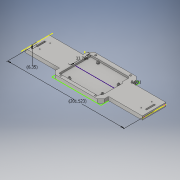
# Autodesk Inventor part: base
Saved by Autodesk Inventor 2016 (Build 200138000, 138)
## iProperties
Created: 2018-02-12
Part Number: base
Material: Generic
Document SubType Name: Modeling
Designer: student
Density: 1 g/cm^3
Appearance: Default
Author: student
Autodesk Inventor part; units mm, degrees
ref_plane "YZ Plane" through (0, 0, 0) normal (1, 0, 0) x (0, 1, 0)
ref_plane "XZ Plane" through (0, 0, 0) normal (0, 1, 0) x (-1, 0, 0)
ref_plane "XY Plane" through (0, 0, 0) normal (0, 0, 1) x (1, 0, 0)
sketch "Sketch1" plane through (0, 0, 0) normal (0, 1, 0) x (-1, 0, 0)
  line L0 (-41.4486, 0) -> (-10.4831, 0)
  line L1 (-10.4831, 0) -> (-10.4831, 53.4636)
  line L2 (-10.4831, 53.4636) -> (-41.4486, 53.4636)
  line L3 (-41.4486, 53.4636) -> (-41.4486, 0)
  line L4 (-79.1688, 53.4636) -> (-87.1698, 53.4636)
  line L5 (-87.1698, 53.4636) -> (-87.1698, 0)
  line L6 (-87.1698, 0) -> (-79.1688, 0)
  line L7 (-79.1688, 0) -> (-79.1688, 53.4636)
  line L8 (-87.1698, 53.4636) -> (-2.487, 53.4636)
  line L9 (-2.487, 53.4636) -> (-2.487, 59.4685)
  line L10 (-2.487, 59.4685) -> (-87.1698, 59.4685)
  line L11 (-87.1698, 59.4685) -> (-87.1698, 53.4636)
  line L12 (-87.1698, 0) -> (-2.487, 0)
  line L13 (-2.487, 0) -> (-2.487, -7.9038)
  line L14 (-2.487, -7.9038) -> (-87.1698, -7.9038)
  line L15 (-87.1698, -7.9038) -> (-87.1698, 0)
  line L16 (-87.1698, -7.9038) -> (-2.487, -7.9038)
  line L17 (-2.487, -7.9038) -> (-2.487, 59.4685)
  line L18 (-2.487, 59.4685) -> (-87.1698, 59.4685)
  line L19 (-87.1698, 59.4685) -> (-87.1698, -7.9038)
  line L20 (-2.487, -7.9038) -> (-2.487, 25.802)
  line L21 (-2.487, 25.802) -> (-2.487, 59.4685)
  point P0 (0, 0)
  dimension "d0" = 8.001
  dimension "d1" = 33.7058
  constraints: 44 end point, 10 parallel, 6 perpendicular, 5 horizontal, 4 point on line
  measures "d0" distance of L6.end L5.end
  measures "d1" distance of L16.end L20.end
extrude "Extrusion1" add sketch "Sketch1" along normal blind 6.35
sketch "Sketch3" plane through (0, 6.35, 0) normal (0, 1, 0) x (1, 0, 0)
  line L0 (10.5148, -0.1125) -> (75.0308, -0.1125) projected
  line L1 (75.0308, -0.1125) -> (76.5548, -1.6365) projected
  line L2 (76.5548, -1.6365) -> (76.5548, -13.003) projected
  line L3 (76.5997, -13.1114) -> (79.0948, -15.6065) projected
  line L4 (79.0948, -15.6065) -> (79.0948, -48.3725) projected
  line L5 (79.0948, -48.3725) -> (76.5997, -50.8676) projected
  line L6 (76.5548, -50.976) -> (76.5548, -53.4525) projected
  line L7 (76.5548, -53.4525) -> (10.5148, -53.4525) projected
  line L8 (10.5148, -53.4525) -> (10.5148, -0.1125) projected
  line L9 (77.3168, -12.7509) -> (77.3168, -1.3209)
  line L10 (77.3168, -1.3209) -> (75.3465, 0.6495)
  line L11 (75.3465, 0.6495) -> (9.7528, 0.6495)
  line L12 (9.7528, 0.6495) -> (9.7528, -54.2145)
  line L13 (9.7528, -54.2145) -> (77.3168, -54.2145)
  line L14 (77.3168, -54.2145) -> (77.3168, -51.2282)
  line L15 (77.3168, -51.2282) -> (79.8568, -48.6882)
  line L16 (79.8568, -48.6882) -> (79.8568, -15.2909)
  line L17 (79.8568, -15.2909) -> (77.3168, -12.7509)
  point P0 (0, 0)
  dimension "d4" = 0.762
  dimension "d5" = 0.762
  dimension "d6" = 0.762
  dimension "d7" = 0.762
  dimension "d8" = 0.762
  dimension "d9" = 0.762
  constraints: 18 end point, 3 other
  measures "d4" distance between parallel lines of L0 L11
  measures "d5" distance between parallel lines of L4 L16
  measures "d6" distance between parallel lines of L15 L5
  measures "d7" distance between parallel lines of L6 L14
  measures "d8" distance between parallel lines of L9 L2
  measures "d9" distance between parallel lines of L3 L17
extrude "Extrusion2" cut sketch "Sketch3" against normal blind 3
sketch "Sketch4" plane through (0, 3.35, 0) normal (0, 1, 0) x (1, 0, 0)
  circle A0 centre (76.5548, -17.8925) radius 1.6 construction
  circle A1 centre (76.5548, -45.8325) radius 1.6 construction
  circle A2 centre (24.4848, -50.9125) radius 1.6 construction
  circle A3 centre (25.7548, -2.6525) radius 1.6 construction
  circle A4 centre (25.7548, -2.6525) radius 2.108
  circle A5 centre (76.5548, -17.8925) radius 2.108
  circle A6 centre (76.5548, -45.8325) radius 2.108
  circle A7 centre (24.4848, -50.9125) radius 2.108
  point P0 (0, 0)
  dimension "d12" = 0.508
  dimension "d13" = 0.508
  dimension "d14" = 0.508
  dimension "d15" = 0.508
  constraints: 4 centre point
  measures "d12" radial gap between concentric circles of A3 A4
  measures "d13" radial gap between concentric circles of A0 A5
  measures "d14" radial gap between concentric circles of A1 A6
  measures "d15" radial gap between concentric circles of A2 A7
extrude "Extrusion3" add sketch "Sketch4" along normal blind 1.1641
sketch "Sketch5" plane through (25.7548, 4.5141, 2.6525) normal (0, 1, 0) x (1, 0, 0)
  circle A0 centre (0, 0) radius 2.108 projected
  circle A1 centre (0, 0) radius 1.6
  circle A2 centre (-1.27, -48.26) radius 2.108 projected
  circle A3 centre (-1.27, -48.26) radius 2.108
  circle A4 centre (-1.27, -48.26) radius 1.6
  circle A5 centre (50.8, -43.18) radius 2.108 projected
  circle A6 centre (50.8, -43.18) radius 2.108
  circle A7 centre (50.8, -15.24) radius 2.108 projected
  circle A8 centre (50.8, -15.24) radius 2.108
  circle A9 centre (50.8, -15.24) radius 1.6
  circle A10 centre (50.8, -43.18) radius 1.6
  point P0 (-25.7548, 2.6525)
  dimension "d18" = 3.2
  dimension "d27" = 3.2
  dimension "d28" = 3.2
  dimension "d29" = 3.2
  constraints: 7 centre point, 4 coincident
  measures "d18" diameter of A1
  measures "d27" diameter of A4
  measures "d28" diameter of A9
  measures "d29" diameter of A10
extrude "Extrusion4" add sketch "Sketch5" along normal blind 1.6002 contours A1 | A4 | A9 | A10
sketch "Sketch8" plane through (25.7548, 6.1143, 2.6525) normal (0, 1, 0) x (1, 0, 0)
  circle A0 centre (0, 0) radius 0.7658
  circle A1 centre (50.8, -15.24) radius 1.6 projected
  circle A2 centre (50.8, -15.24) radius 0.7658
  circle A3 centre (50.8, -43.18) radius 1.6 projected
  circle A4 centre (50.8, -43.18) radius 0.7658
  circle A5 centre (-1.27, -48.26) radius 1.6 projected
  circle A6 centre (-1.27, -48.26) radius 0.7658
  point P0 (-25.7548, 2.6525)
  dimension "d32" = 1.5316
  dimension "d33" = 1.5316
  dimension "d34" = 1.5316
  dimension "d35" = 1.5316
  constraints: 4 centre point, 3 coincident
  measures "d32" diameter of A0
  measures "d33" diameter of A2
  measures "d34" diameter of A4
  measures "d35" diameter of A6
extrude "Extrusion5" cut sketch "Sketch8" against normal blind 14.986 contours A0 | A2 | A4 | A6
sketch "Sketch9" plane through (0, 6.35, 0) normal (0, 1, 0) x (1, 0, 0)
  line L0 (87.1698, 7.9038) -> (2.487, 7.9038) projected
  line L1 (44.8284, 7.9038) -> (44.8284, -59.4685)
  line L2 (2.487, -59.4685) -> (87.1698, -59.4685) projected
  line L3 (2.487, 7.9038) -> (2.487, -59.4685) projected
  line L4 (2.487, -25.7823) -> (87.1698, -25.7823)
  line L5 (87.1698, -59.4685) -> (87.1698, 7.9038) projected
  line L6 (2.487, -25.7823) -> (-55.933, -25.7823)
  line L7 (-55.933, -25.7823) -> (-55.933, -5.4623)
  line L8 (-55.933, -5.4623) -> (2.487, -5.4623)
  line L9 (2.487, -5.4623) -> (2.487, -25.7823)
  line L10 (-55.933, -25.7823) -> (-55.933, -46.1023)
  line L11 (-55.933, -46.1023) -> (2.487, -46.1023)
  circle A0 centre (14.7725, 4.3917) radius 1.524
  line L12 (145.5898, -25.7823) -> (145.5898, -5.4623)
  line L13 (145.5898, -5.4623) -> (87.1698, -5.4623)
  line L14 (145.5898, -25.7823) -> (145.5898, -46.1023)
  line L15 (145.5898, -46.1023) -> (87.1698, -46.1023)
  circle A1 centre (74.8844, 4.3917) radius 1.524
  circle A2 centre (14.7725, -55.9564) radius 1.524
  circle A3 centre (74.8844, -55.9564) radius 1.524
  line L16 (87.1698, -46.1023) -> (87.1698, -5.4623)
  line L17 (2.487, -46.1023) -> (2.487, -5.4623)
  circle A4 centre (14.7725, -55.9564) radius 1.524
  circle A5 centre (14.7725, 4.3917) radius 1.524
  circle A6 centre (74.8844, 4.3917) radius 1.524
  point P0 (0, 0)
  dimension "d38" = 58.42
  dimension "d39" = 20.32
  dimension "d40" = 3.048
  constraints: 28 end point, 10 symmetric about line, 7 centre point, 4 midpoint, 3 coincident, 3 concentric, 2 parallel, 2 perpendicular, 1 collinear, 1 horizontal, 3 other
  measures "d38" distance of L7.end L8.end
  measures "d39" distance of L6.end L7.end
  measures "d40" diameter of A0
extrude "Extrusion6" add sketch "Sketch9" against normal blind 6.35 contours L13 L12 L14 L15 L5 | L3 L6 L7 L8 | L3 L11 L10 L6
sketch "Sketch10" plane through (0, 6.35, 0) normal (0, 1, 0) x (1, 0, 0)
  point P0 (0, 0)
extrude "Extrusion7" cut sketch "Sketch9" against normal blind 9.906 contours A0 | A1 | A2 | A3
sketch "Sketch11" plane through (0, 6.35, 0) normal (0, 1, 0) x (1, 0, 0)
  line L0 (-55.933, -46.1023) -> (-55.933, -5.4623) projected
  line L1 (-55.933, -25.7823) -> (145.5898, -25.7823)
  line L2 (145.5898, -5.4623) -> (145.5898, -46.1023) projected
  line L3 (87.1698, 7.9038) -> (2.487, 7.9038) projected
  line L4 (44.8284, 7.9038) -> (44.8284, -59.4685)
  line L5 (2.487, -59.4685) -> (87.1698, -59.4685) projected
  line L6 (-55.933, -25.7823) -> (-26.469, -25.7823)
  line L7 (-26.469, -25.7823) -> (-26.469, -19.5593)
  line L8 (-26.469, -19.5593) -> (-55.933, -19.5593)
  line L9 (-55.933, -19.5593) -> (-55.933, -25.7823)
  line L10 (-26.469, -25.7823) -> (-55.933, -25.7823)
  line L11 (-55.933, -25.7823) -> (-55.933, -32.0067)
  line L12 (-55.933, -32.0067) -> (-26.469, -32.0067)
  line L13 (-26.469, -32.0067) -> (-26.469, -25.7823)
  line L14 (-55.933, -25.7823) -> (-26.469, -25.7823)
  line L15 (-26.469, -25.7823) -> (-26.469, -32.0067)
  line L16 (-26.469, -32.0067) -> (-55.933, -32.0067)
  line L17 (-55.933, -32.0067) -> (-55.933, -25.7823)
  line L18 (-55.933, -19.5593) -> (-38.633, -19.5593)
  line L19 (-55.933, -25.7823) -> (-55.933, -18.2823)
  line L20 (-55.933, -18.2823) -> (-38.633, -18.2823)
  line L21 (-38.633, -18.2823) -> (-38.633, -12.4823)
  line L22 (-38.633, -12.4823) -> (-47.133, -12.4823)
  line L23 (-47.133, -12.4823) -> (-47.133, -18.2823)
  line L24 (-48.3704, -25.7823) -> (-48.3704, -18.1623)
  line L25 (-48.3704, -18.1623) -> (-50.9104, -18.1623)
  line L26 (-50.9104, -18.1623) -> (-50.9104, -25.7823)
  line L27 (-42.883, -25.7823) -> (-42.883, -16.7823)
  circle A0 centre (-42.883, -16.7823) radius 0.8001
  line L28 (-48.3704, -25.7823) -> (-48.3704, -33.4023)
  line L29 (-48.3704, -33.4023) -> (-50.9104, -33.4023)
  line L30 (-50.9104, -33.4023) -> (-50.9104, -25.7823)
  circle A1 centre (-42.883, -34.7823) radius 0.8001
  line L31 (138.0273, -25.7823) -> (138.0273, -18.1623)
  line L32 (138.0273, -18.1623) -> (140.5673, -18.1623)
  line L33 (140.5673, -18.1623) -> (140.5673, -25.7823)
  circle A2 centre (132.5398, -16.7823) radius 0.8001
  circle A3 centre (132.5398, -34.7823) radius 0.8001
  line L34 (138.0273, -25.7823) -> (138.0273, -33.4023)
  line L35 (140.5673, -33.4023) -> (140.5673, -25.7823)
  line L36 (138.0273, -33.4023) -> (140.5673, -33.4023)
  point P0 (0, 0)
  dimension "d64" = 2
  dimension "d45" = 29.464
  dimension "d46" = 6.223
  dimension "d47" = 17.3
  dimension "d48" = 7.5
  dimension "d49" = 5.8
  dimension "d50" = 8.5
  dimension "d51" = 7.62
  dimension "d52" = 2.54
  dimension "d53" = 9
  dimension "d54" = 1.6002
  constraints: 66 end point, 11 symmetric about line, 9 parallel, 8 perpendicular, 7 point on line, 4 centre point, 4 midpoint, 3 horizontal, 1 coincident, 3 other
  measures "d45" distance of L8.end L7.end
  measures "d46" distance of L7.end L6.end
  measures "d47" distance of L8.end L18.end
  measures "d48" distance of L10.end L19.end
  measures "d49" distance of L20.end L21.end
  measures "d50" distance of L21.end L22.end
  measures "d51" distance of L24.start L24.end
  measures "d52" distance of L24.end L25.end
  measures "d53" distance of L27.start L27.end
  measures "d54" diameter of A0
extrude "Extrusion8" cut sketch "Sketch11" against normal blind 25.4 contours L31 L32 L33 L1 | L1 L35 L36 L34 | L30 L1 L28 L12 | L12 L28 L29 L30 | L26 L8 L24 L1 | L26 L20 L24 L8 | L26 L25 L24 L20 | A0 | A1 | A2 | A3
sketch "Sketch12" plane through (87.1698, 0, -7.9038) normal (0, 0, -1) x (-1, 0, 0)
  point P0 (87.1698, 0)
sketch "Sketch13" plane through (-55.933, 6.35, 8.6373) normal (-1, 0, 0) x (0, 0, 1)
  point P0 (-8.6373, -6.35)
sketch "Sketch15" plane through (0, 3.35, 0) normal (0, 1, 0) x (1, 0, 0)
  line L0 (-55.933, -5.4623) -> (-55.933, -46.1023) projected
  line L1 (-55.933, -25.7823) -> (145.5898, -25.7823)
  line L2 (145.5898, -5.4623) -> (145.5898, -46.1023) projected
  point P0 (0, 0)
  point P1 (-55.933, -8.6373)
  point P2 (-55.933, -42.9273)
  point P3 (145.5898, -8.6373)
  point P4 (145.5898, -42.9273)
  dimension "d61" = 201.5228
  constraints: 2 end point, 2 midpoint
  measures "d61" distance of L1.start L1.end
sketch "Sketch16" plane through (-55.933, 6.35, 8.6373) normal (-1, 0, 0) x (0, 0, 1)
  line L0 (45.5772, 0) -> (-9.2868, 0) projected
  line L1 (18.1452, 0) -> (18.1452, -6.35)
  line L2 (9.525, -6.35) -> (24.765, -6.35) projected
  point P0 (-8.6373, -6.35)
  dimension "d62" = 6.35
  constraints: 2 end point, 1 midpoint, 1 point on line, 1 vertical
  measures "d62" distance of L1.start L1.end
chamfer "Chamfer2" distance 6 angle 45 4 edges at (87.1698, 3.175, -7.9038) (87.1698, 3.175, 59.4685) (2.487, 3.175, 59.4685) (2.487, 3.175, -7.9038)
equation "\"d4\" = d5"
equation "\"d6\" = d5"
equation "\"d7\" = d5"
equation "\"d8\" = d5"
equation "\"d9\" = d5"
equation "\"d13\" = d12"
equation "\"d14\" = d12"
equation "\"d15\" = d12"
body "Solid1"
